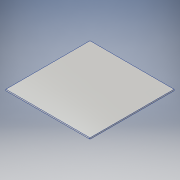
# Autodesk Inventor part: Turntable Bottom
Saved by Autodesk Inventor 2016 (Build 200138000, 138)
## iProperties
Created: 2018-05-16
Part Number: Turntable Bottom
Material: Aluminum 6061
Document SubType Name: Modeling
Designer: Kade
Density: 2.7 g/cm^3
Appearance: Aluminum - Flat
Mass: 353.961 g
Surface Area: 851.611 cm^2
Volume: 131.097 cm^3
Author: Kade
Autodesk Inventor part; units mm, degrees
ref_plane "YZ Plane" through (0, 0, 0) normal (1, 0, 0) x (0, 1, 0)
ref_plane "XZ Plane" through (0, 0, 0) normal (0, 1, 0) x (-1, 0, 0)
ref_plane "XY Plane" through (0, 0, 0) normal (0, 0, 1) x (1, 0, 0)
sketch "Sketch1" plane through (0, 0, 0) normal (0, 1, 0) x (-1, 0, 0)
  line L0 (-101.6, 101.6) -> (101.6, 101.6)
  line L1 (101.6, 101.6) -> (101.6, -101.6)
  line L2 (101.6, -101.6) -> (-101.6, -101.6)
  line L3 (-101.6, -101.6) -> (-101.6, 101.6)
  line L4 (-101.6, 101.6) -> (101.6, -101.6) construction
  line L5 (101.6, 101.6) -> (-101.6, -101.6) construction
  point P0 (0, 0)
  dimension "d0" = 203.2
  dimension "d1" = 203.2
  constraints: 12 end point, 2 midpoint, 2 parallel, 1 horizontal, 1 perpendicular
  measures "d0" distance of L1.end L2.end
  measures "d1" distance of L0.end L1.end
extrude "Extrusion1" add sketch "Sketch1" along normal blind 3.175
body "Solid1"
